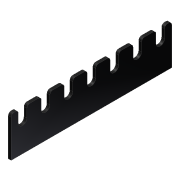
# Autodesk Inventor part: Belt_CombGuide_Intake
Saved by Autodesk Inventor 2012 (Build 160160000, 160)
## iProperties
Created: 2012-01-25
Part Number: Belt_CombGuide_Intake
Material: Default
Document SubType Name: Modeling
Designer: JesseK
Density: 1 g/cm^3
Mass: 21.5025 g
Surface Area: 155.723 cm^2
Volume: 21.5025 cm^3
Author: JesseK
Autodesk Inventor part; units mm, degrees
ref_plane "YZ Plane" through (0, 0, 0) normal (1, 0, 0) x (0, 1, 0)
ref_plane "XZ Plane" through (0, 0, 0) normal (0, 1, 0) x (-1, 0, 0)
ref_plane "XY Plane" through (0, 0, 0) normal (0, 0, 1) x (1, 0, 0)
sketch "Sketch1" plane through (0, 0, 0) normal (0, 0, 1) x (1, 0, 0)
  line L0 (0, 0) -> (3.175, 0)
  line L1 (3.175, 0) -> (3.175, 44.45)
  line L2 (3.175, 44.45) -> (0, 44.45)
  line L3 (0, 44.45) -> (0, 0)
  dimension "d0" = 44.45
  dimension "d18" = 3.175
  constraints: 8 end point, 2 horizontal, 2 vertical
  measures "d0" distance of L2.end L0.start
  measures "d18" distance between parallel lines of L3 L1
extrude "Extrusion1" add sketch "Sketch1" along normal blind 177.8
sketch "Sketch3" plane through (0, 0, 0) normal (-1, 0, 0) x (0, 0, 1)
  line L0 (0, 44.45) -> (177.8, 44.45) projected
  line L1 (0, 44.45) -> (0, 0) projected
  line L2 (7.9375, 44.45) -> (7.9375, 31.75)
  line L3 (17.4625, 31.75) -> (17.4625, 44.45)
  arc A0 (7.9375, 31.75) -> (17.4625, 31.75) centre (12.7, 31.75) ccw
  line L4 (7.9375, 44.45) -> (17.4625, 44.45)
  dimension "d9" = 9.525
  dimension "d10" = 12.7
  dimension "d11" = 12.7
  constraints: 6 end point, 2 point on circle, 2 point on line, 2 tangent, 2 vertical, 1 centre point, 1 horizontal
  measures "d9" distance between parallel lines of L3 L2
  measures "d10" distance of L2.start L2.end
  measures "d11" distance from line of L1 A0.centre
extrude "Extrusion3" cut sketch "Sketch3" against normal through all
pattern_linear "Rectangular Pattern1" count 7 spacing 25.4 along (0, 0, 1) of "Extrusion3"
fillet "Fillet1" radius 3.175 16 edges at (1.5875, 44.45, 177.8) (1.5875, 44.45, 169.8625) (1.5875, 44.45, 160.3375) (1.5875, 44.45, 144.4625) (1.5875, 44.45, 134.9375) (1.5875, 44.45, 119.0625) (1.5875, 44.45, 109.5375) (1.5875, 44.45, 93.6625) (1.5875, 44.45, 84.1375) (1.5875, 44.45, 68.2625) (1.5875, 44.45, 58.7375) (1.5875, 44.45, 42.8625) (1.5875, 44.45, 33.3375) (1.5875, 44.45, 17.4625) (1.5875, 44.45, 7.9375) (1.5875, 44.45, 0)
body "Solid1"
